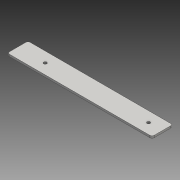
# Autodesk Inventor part: extension3
Saved by Autodesk Inventor 2016 (Build 200138000, 138)
## iProperties
Created: 2019-01-31
Part Number: extension3
Material: Generic
Document SubType Name: Modeling
Designer: TYP
Density: 1 g/cm^3
Appearance: Default
Author: TYP
Autodesk Inventor part; units mm, degrees
ref_plane "YZ Plane" through (0, 0, 0) normal (1, 0, 0) x (0, 1, 0)
ref_plane "XZ Plane" through (0, 0, 0) normal (0, 1, 0) x (-1, 0, 0)
ref_plane "XY Plane" through (0, 0, 0) normal (0, 0, 1) x (1, 0, 0)
sketch "Sketch1" plane through (0, 0, 0) normal (0, 0, 1) x (1, 0, 0)
  line L0 (-105, -15) -> (105, -15)
  line L1 (105, -15) -> (105, 15)
  line L2 (105, 15) -> (-105, 15)
  line L3 (-105, 15) -> (-105, -15)
  line L4 (-105, -15) -> (105, 15) construction
  line L5 (105, -15) -> (-105, 15) construction
  circle A0 centre (85, 0) radius 2.25
  circle A1 centre (-65, 0) radius 2.25
  point P0 (0, 0)
  point P1 (0, 0)
  point P2 (0, 0)
  dimension "d0" = 210
  dimension "d1" = 30
  dimension "d2" = 4.5
  dimension "d3" = 4.5
  dimension "d4" = 20
  dimension "d5" = 150
  constraints: 12 end point, 4 midpoint, 2 centre point, 2 horizontal alignment, 2 parallel, 1 horizontal, 1 perpendicular
  measures "d0" distance of L2.end L1.end
  measures "d1" distance of L1.end L0.end
  measures "d2" diameter of A0
  measures "d3" diameter of A1
  measures "d4" distance from line of L1 A0.centre
  measures "d5" distance of A1.centre A0.centre
extrude "Extrusion1" add sketch "Sketch1" along normal blind 3
fillet "Fillet1" radius 3 4 edges at (105, -15, 1.5) (105, 15, 1.5) (-105, 15, 1.5) (-105, -15, 1.5)
body "Solid1"
